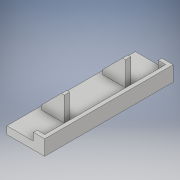
# Autodesk Inventor part: MonsterHolder
Saved by Autodesk Inventor 2019 (Build 230136000, 136)
## iProperties
Created: 2018-12-03
Part Number: MonsterHolder
Material: Generic
Document SubType Name: Modeling
Designer: Administrator
Density: 1 g/cm^3
Appearance: Default
Author: Administrator
Autodesk Inventor part; units mm, degrees
ref_plane "YZ Plane" through (0, 0, 0) normal (1, 0, 0) x (0, 1, 0)
ref_plane "XZ Plane" through (0, 0, 0) normal (0, 1, 0) x (-1, 0, 0)
ref_plane "XY Plane" through (0, 0, 0) normal (0, 0, 1) x (1, 0, 0)
sketch "Sketch1" plane through (0, 0, 0) normal (1, 0, 0) x (0, 1, 0)
  line L0 (0, 0) -> (38.1, 0)
  line L1 (38.1, 0) -> (38.1, -101.6)
  line L2 (38.1, -101.6) -> (0, -101.6)
  line L3 (0, -101.6) -> (0, 0)
  dimension "d0" = 101.6
  dimension "d1" = 38.1
  constraints: 8 end point, 2 parallel, 1 horizontal, 1 perpendicular
  measures "d0" distance of L0.end L1.end
  measures "d1" distance of L0.start L0.end
extrude "Extrusion1" add sketch "Sketch1" along normal blind 6.35
sketch "Sketch2" plane through (0, 0, 0) normal (-1, 0, 0) x (0, 0, 1)
  line L0 (0, 0) -> (0, 38.1) projected
  line L1 (-101.6, 38.1) -> (-101.6, 0) projected
  line L2 (-101.6, 0) -> (0, 0) projected
  line L3 (0, 0) -> (-101.6, 0) projected
  line L4 (-78.74, 0) -> (-74.295, 0)
  line L5 (-74.295, 0) -> (-74.295, 20.32)
  line L6 (-74.295, 20.32) -> (-78.74, 20.32)
  line L7 (-78.74, 20.32) -> (-78.74, 0)
  line L8 (-27.305, 0) -> (-22.86, 0)
  line L9 (-22.86, 0) -> (-22.86, 20.32)
  line L10 (-22.86, 20.32) -> (-27.305, 20.32)
  line L11 (-27.305, 20.32) -> (-27.305, 0)
  dimension "d10" = 4.445
  dimension "d11" = 4.445
  dimension "d13" = 20.32
  dimension "d14" = 22.86
  dimension "d15" = 22.86
  constraints: 16 end point, 4 parallel, 3 point on line, 2 horizontal, 2 perpendicular
  measures "d10" distance of L9.end L10.end
  measures "d11" distance of L5.end L6.end
  measures "d13" distance of L6.end L4.start
  measures "d14" distance between parallel lines of L1 L7
  measures "d15" distance between parallel lines of L0 L9
extrude "Extrusion2" add sketch "Sketch2" along normal blind 19.05
chamfer "Chamfer1" distance 16.51 angle 45 2 edges at (-19.05, 20.32, -25.0825) (-19.05, 20.32, -76.5175)
sketch "Sketch3" plane through (0, 0, -101.6) normal (0, -1, 0) x (1, 0, 0)
  line L0 (0, 0) -> (6.35, 0) projected
  line L1 (9.525, -3.175) -> (-22.225, -3.175)
  line L2 (0, 101.6) -> (6.35, 101.6) projected
  line L3 (9.525, -3.175) -> (9.525, 104.775)
  line L4 (9.525, 104.775) -> (-22.225, 104.775)
  line L5 (-22.225, -3.175) -> (-22.225, 104.775)
  line L6 (-19.05, 22.86) -> (-19.05, 27.305) projected
  line L7 (6.35, 101.6) -> (6.35, 0) projected
  dimension "d22" = 3.175
  dimension "d25" = 3.175
  dimension "d26" = 3.175
  dimension "d27" = 3.175
  dimension "d52" = 107.95
  dimension "d53" = 31.75
  constraints: 8 end point, 2 perpendicular, 1 horizontal, 1 vertical
  measures "d22" distance between parallel lines of L1 L0
  measures "d25" distance between parallel lines of L2 L4
  measures "d26" distance between parallel lines of L5 L6
  measures "d27" distance between parallel lines of L3 L7
  measures "d52" distance between parallel lines of L1 L4
  measures "d53" distance of L1.start L1.end
extrude "Extrusion3" add sketch "Sketch3" along normal blind 6.35
sketch "Sketch4" plane through (0, 0, -101.6) normal (0, 1, 0) x (1, 0, 0)
  line L0 (0, -101.6) -> (6.35, -101.6) projected
  line L1 (0, -101.6) -> (6.35, -101.6)
  line L2 (6.35, -101.6) -> (6.35, 0) projected
  line L3 (6.35, -101.6) -> (6.35, 0)
  line L4 (6.35, 0) -> (0, 0)
  line L5 (0, 0) -> (0, 3.175)
  line L6 (9.525, 3.175) -> (-22.225, 3.175) projected
  line L7 (0, 3.175) -> (9.525, 3.175)
  line L8 (9.525, 3.175) -> (9.525, -104.775) projected
  line L9 (9.525, 3.175) -> (9.525, -104.775)
  line L10 (9.525, -104.775) -> (0, -104.775)
  line L11 (-22.225, -104.775) -> (9.525, -104.775) projected
  line L12 (0, -104.775) -> (0, -101.6)
  constraints: 16 end point, 4 perpendicular, 3 point on line, 2 collinear, 1 horizontal
extrude "Extrusion5" add sketch "Sketch4" along normal blind 6.35
sketch "Sketch5" plane through (0, 38.1, 0) normal (0, 1, 0) x (1, 0, 0)
  line L0 (0, 0) -> (0, -3.175) projected
  line L1 (0, 0) -> (6.35, 0)
  line L2 (6.35, 0) -> (6.35, 101.6)
  line L3 (6.35, 101.6) -> (0, 101.6)
  line L4 (0, 101.6) -> (0, 0)
  constraints: 8 end point, 2 parallel, 1 horizontal, 1 perpendicular
extrude "Extrusion6" cut sketch "Sketch5" against normal blind 38.1
body "Solid1"
